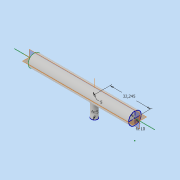
# Autodesk Inventor part: lw_5_цилиндр
Saved by Autodesk Inventor 2019 (Build 230136000, 136)
## iProperties
Created: 2021-04-29
Part Number: lw_5_цилиндр
Material: Типовые
Document SubType Name: Modeling
Designer: Kurbatova
Density: 1 g/cm^3
Appearance: По умолчанию
diametr_: 10,000 мм
diametr_ruchka_: 5,000 мм
length: 80,000 мм
Author: Kurbatova
Autodesk Inventor part; units mm, degrees
ref_plane "YZ Plane" through (0, 0, 0) normal (1, 0, 0) x (0, 1, 0)
ref_plane "XZ Plane" through (0, 0, 0) normal (0, 1, 0) x (-1, 0, 0)
sketch "цилиндр_конец1" plane through (0, 0, 0) normal (1, 0, 0) x (0, 1, 0)
  line L0 (5, 0) -> (-5, 0)
  line L1 (0, 5) -> (0, -5)
  circle A0 centre (0, 0) radius 5
  dimension "diametr" = 10
  constraints: 4 end point, 4 point on circle, 2 midpoint, 1 centre point, 1 coincident, 1 horizontal, 1 vertical
  measures "diametr" diameter of A0
extrude "Выдавливание1" add sketch "цилиндр_конец1" against normal blind 80
sketch "цилиндр_конец2" plane through (-80, 0, 0) normal (-1, 0, 0) x (0, 0, 1)
  circle A0 centre (0, 0) radius 5 projected
ref_plane "РабПлоскость7" through (0, 0, 0) normal (0, 1, 0) x (-1, 0, 0)
ref_plane "РабПлоскость8" through (0, 0, 0) normal (0, 0, -1) x (-1, 0, 0)
sketch "ручка_конец1" plane through (0, 0, 0) normal (0, 1, 0) x (-1, 0, 0)
  line L0 (0, 5) -> (0, -5) projected
  line L1 (80, -5) -> (80, 5) projected
  circle A0 centre (32.245, 0) radius 2.5
  line L2 (-16, 0) -> (96, 0) projected
  point P0 (0, 0)
  dimension "d43" = 5
  dimension "d44" = 32.245
  constraints: 1 centre point, 1 point on line
  measures "d43" diameter of A0
  measures "d44" distance from line of A0.centre L0
ref_plane "РабПлоскость9" through (0, -15.61, 0) normal (0, 1, 0) x (-1, 0, 0)
sketch "ручка_конец2" plane through (0, -15.61, 0) normal (0, 1, 0) x (-1, 0, 0)
  circle A0 centre (32.245, 0) radius 2.5
  point P0 (0, 0)
  dimension "diametr_ruchka" = 5
  constraints: 1 centre point, 1 coincident
  measures "diametr_ruchka" diameter of A0
loft "Лофт1" add profiles "ручка_конец1", "ручка_конец2"
equation "\"diametr\" = diametr_"
equation "\"d1\" = length"
equation "\"diametr_ruchka\" = diametr_ruchka_"
equation "\"diametr_\" = 10"
equation "\"diametr_ruchka_\" = 5"
equation "\"length\" = 80"
